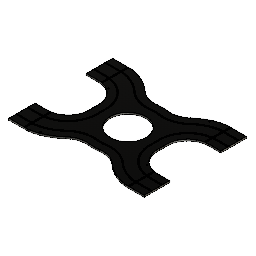
_10-16 (Round-about).bfac9250-3655-4f17-af9d-ce13ce2a29ba (Autodesk Fusion 360 design; units mm, degrees)
Autodesk Fusion 360 part; units mm, degrees
note: some values were not read from the file. Set by a fixed rule: which sketch regions a step uses.
sketch "Sketch1" plane through (0, 0, 0) normal (0, 0, 1) x (1, 0, 0)
  line L0 (0, 0) -> (609.6, 0)
  line L1 (609.6, 0) -> (609.6, -838.2)
  line L2 (609.6, -838.2) -> (0, -838.2)
  line L3 (0, -838.2) -> (0, 0)
  line L4 (0, -838.2) -> (0, -2438.4)
  line L5 (0, -2438.4) -> (609.6, -2438.4)
  line L6 (609.6, -2438.4) -> (609.6, -3276.6)
  line L7 (609.6, -3276.6) -> (0, -3276.6)
  line L8 (0, -3276.6) -> (0, -2438.4)
  line L9 (609.6, -838.2) -> (609.6, -1638.3)
  line L10 (609.6, -1638.3) -> (1036.4572, -1638.3)
  circle A0 centre (2120.9, -1638.3) radius 1084.4428
  circle A1 centre (2120.9, -1638.3) radius 558.8
  line L11 (2120.9, -1638.3) -> (3205.3428, -1638.3)
  line L12 (3205.3428, -1638.3) -> (3632.2, -1638.3)
  line L13 (2120.9, -1638.3) -> (1036.4572, -1638.3)
  line L14 (3632.2, -25.4) -> (4241.8, -25.4)
  line L15 (4241.8, -25.4) -> (4241.8, -838.2)
  line L16 (4241.8, -838.2) -> (3632.2, -838.2)
  line L17 (3632.2, -838.2) -> (3632.2, -25.4)
  line L18 (3632.2, -838.2) -> (3632.2, -2438.4)
  line L19 (3632.2, -2438.4) -> (4241.8, -2438.4)
  line L20 (4241.8, -2438.4) -> (4241.8, -3251.2)
  line L21 (4241.8, -3251.2) -> (3632.2, -3251.2)
  line L22 (3632.2, -3251.2) -> (3632.2, -2438.4)
  circle A2 centre (381.6587, -1498.6) radius 660.4
  circle A3 centre (381.6587, -1778) radius 660.4
  circle A4 centre (381.6587, -1778) radius 1515.8361
  circle A5 centre (1870.653, -3365.1042) radius 660.4
  circle A6 centre (3860.1413, -1778) radius 660.4
  circle A7 centre (3860.1413, -1498.6) radius 660.4
  circle A8 centre (3860.1413, -1778) radius 1490.7298
  circle A9 centre (2402.7721, -3360.2246) radius 660.4
  circle A10 centre (381.6587, -1498.6) radius 1515.8361
  circle A11 centre (3860.1413, -1498.6) radius 1490.7298
  circle A12 centre (1870.653, 88.5042) radius 660.4
  circle A13 centre (2402.7721, 83.6246) radius 660.4
  point P0 (3632.2, -1638.3)
  point P1 (3632.2, -1638.3)
  dimension "d1" = 609.6
  dimension "d2" = 838.2
  dimension "d3" = 1600.2
  dimension "d4" = 609.6
  dimension "d5" = 838.2
  dimension "d9" = 1117.6
  dimension "d24" = 609.6
  dimension "d36" = 1320.8
  dimension "d37" = 1320.8
  dimension "d38" = 1320.8
  dimension "d39" = 1320.8
  dimension "d40" = 1320.8
  dimension "d41" = 1320.8
  constraint horizontal L0
  constraint vertical L1
  constraint horizontal L2
  constraint vertical L3
  constraint coincident L0.start L3.end
  constraint perpendicular L2 L4
  constraint horizontal L5
  constraint vertical L6
  constraint horizontal L7
  constraint vertical L8
  constraint perpendicular L5 L9
  constraint perpendicular L9 L10
  constraint coincident L10.end A0
  constraint concentric A0 A1
  constraint coincident A0.centre A1.centre
  constraint coincident A0 L11.end
  constraint horizontal L11
  constraint parallel L11 L12
  constraint parallel L10 L13
  constraint horizontal L14
  constraint vertical L15
  constraint horizontal L16
  constraint vertical L17
  constraint perpendicular L16 L18
  constraint horizontal L19
  constraint vertical L20
  constraint horizontal L21
  constraint vertical L22
  constraint midpoint L18 P1
  constraint tangent L2 A2
  constraint tangent A0 A2
  constraint tangent A0 A3
  constraint tangent L5 A3
  constraint concentric A3 A4
  constraint coincident L6.end A4
  constraint tangent A4 A5
  constraint tangent A0 A5
  constraint tangent A0 A6
  constraint tangent L19 A6
  constraint tangent A0 A7
  constraint tangent L16 A7
  constraint concentric A6 A8
  constraint coincident L21.end A8
  constraint tangent A0 A9
  constraint tangent A8 A9
  constraint concentric A2 A10
  constraint coincident L0.end A10
  constraint concentric A7 A11
  constraint coincident L14.start A11
  constraint symmetric L11 A5 A12
  constraint symmetric L11 A9 A13
  measures "d1" distance of L0.start L0.end
  measures "d2" distance of L0.start L2.end
  measures "d3" distance of L2.end L4.end
  measures "d4" distance of L4.end L5.end
  measures "d5" distance of L4.end L7.end
  measures "d9" diameter of A1
  measures "d24" distance of L14.start L14.end
  measures "d36" diameter of A2
  measures "d37" diameter of A3
  measures "d38" diameter of A5
  measures "d39" diameter of A6
  measures "d40" diameter of A7
  measures "d41" diameter of A9
extrude "Extrude2" add sketch "Sketch1" along normal blind 50.8 contours L0 L3 A10 | L0 L1 L3 A4 A10 | L1 A0 A4 A10 | L1 L2 L3 A4 | L1 L9 A0 A2 A4 | A0 A10 A12 | L7 L8 A4 | L6 L7 L8 A4 A10 | L5 L6 L8 A10 | L2 L9 A2 | A0 A1 L13 A4 | A0 A1 A4 A10 | A0 A1 A10 A11 | L6 A0 A4 A10 | L5 L6 A0 A3 A10 | A0 A11 A13 | A0 A1 A4 A10 | A0 A1 L13 A10 | A0 A1 A8 A11 | A0 L17 A8 A11 | A0 A4 A5 | A0 A1 A4 A8 | A0 A1 L11 A8 | L14 L15 L17 A8 A11 | A0 L17 L18 A7 A8 | A0 A1 L11 A11 | A0 A1 A8 A11 | L14 L15 A11 | L15 L16 L17 A8 | A0 A8 A9 | A0 L22 A8 A11 | A0 L18 L22 A6 A11 | L16 L18 A7 | L20 L21 L22 A8 A11 | L19 L20 L22 A11 | L18 L19 A6 | L20 L21 A8
sketch "Sketch2" plane through (0, 0, 0) normal (0, 0, -1) x (1, 0, 0)
  circle A0 centre (2120.9, 1638.3) radius 558.8
  arc A1 (1418.8032, 2883.482) -> (609.6, 3276.6) centre (381.6587, 1778) ccw
  line L0 (609.6, 3276.6) -> (0, 3276.6)
  line L1 (0, 3276.6) -> (0, 2438.4)
  line L2 (0, 2438.4) -> (381.6587, 2438.4)
  arc A2 (1039.9386, 1725.1254) -> (381.6587, 2438.4) centre (381.6587, 1778) ccw
  arc A3 (1039.9386, 1725.1254) -> (1039.9386, 1551.4746) centre (2120.9, 1638.3) ccw
  arc A4 (381.6587, 838.2) -> (1039.9386, 1551.4746) centre (381.6587, 1498.6) ccw
  line L3 (381.6587, 838.2) -> (0, 838.2)
  line L4 (0, 838.2) -> (0, 0)
  line L5 (0, 0) -> (609.6, 0)
  arc A5 (609.6, 0) -> (1418.8032, 393.118) centre (381.6587, 1498.6) ccw
  arc A6 (1965.3682, 565.0685) -> (1418.8032, 393.118) centre (1870.653, -88.5042) ccw
  arc A7 (1965.3682, 565.0685) -> (2296.0872, 568.1012) centre (2120.9, 1638.3) ccw
  arc A8 (2850.1866, 402.1207) -> (2296.0872, 568.1012) centre (2402.7721, -83.6246) ccw
  arc A9 (2850.1866, 402.1207) -> (3632.2, 25.4) centre (3860.1413, 1498.6) ccw
  line L6 (3632.2, 25.4) -> (4241.8, 25.4)
  line L7 (4241.8, 25.4) -> (4241.8, 838.2)
  line L8 (4241.8, 838.2) -> (3860.1413, 838.2)
  arc A10 (3201.8614, 1551.4746) -> (3860.1413, 838.2) centre (3860.1413, 1498.6) ccw
  arc A11 (3201.8614, 1551.4746) -> (3201.8614, 1725.1254) centre (2120.9, 1638.3) ccw
  arc A12 (3860.1413, 2438.4) -> (3201.8614, 1725.1254) centre (3860.1413, 1778) ccw
  line L9 (3860.1413, 2438.4) -> (4241.8, 2438.4)
  line L10 (4241.8, 2438.4) -> (4241.8, 3251.2)
  line L11 (4241.8, 3251.2) -> (3632.2, 3251.2)
  arc A13 (3632.2, 3251.2) -> (2850.1866, 2874.4793) centre (3860.1413, 1778) ccw
  arc A14 (2296.0872, 2708.4988) -> (2850.1866, 2874.4793) centre (2402.7721, 3360.2246) ccw
  arc A15 (2296.0872, 2708.4988) -> (1965.3682, 2711.5315) centre (2120.9, 1638.3) ccw
  arc A16 (1418.8032, 2883.482) -> (1965.3682, 2711.5315) centre (1870.653, 3365.1042) ccw
  line L12 (198.4059, 2636.3069) -> (672.8085, 2636.3069) construction
  line L13 (672.8085, 2636.3069) -> (672.8085, 3106.5481) construction
  line L14 (672.8085, 3106.5481) -> (198.4059, 3106.5481) construction
  line L15 (198.4059, 3106.5481) -> (198.4059, 2636.3069) construction
  line L16 (0, 508) -> (482.6, 508)
  line L17 (0, 2794) -> (482.6, 2794)
  line L18 (4241.8, 272.4179) -> (3759.2, 272.4179)
  line L19 (4241.8, 2844.8) -> (3759.2, 2844.8)
  line L20 (482.6, 508) -> (482.6, 0)
  line L21 (3759.2, 272.4179) -> (3759.2, 845.96)
  line L22 (3759.2, 2844.8) -> (3759.2, 2430.64)
  line L23 (482.6, 2794) -> (482.6, 2430.64)
  line L24 (482.6, 2430.64) -> (511.175, 2430.64)
  line L25 (511.175, 2430.64) -> (511.175, 3276.6)
  line L26 (511.175, 3276.6) -> (482.6, 3276.6)
  line L27 (482.6, 3276.6) -> (482.6, 2430.64)
  line L28 (482.6, 0) -> (511.175, 0)
  line L29 (511.175, 0) -> (511.175, 851.0248)
  line L30 (511.175, 851.0248) -> (482.6, 851.0248)
  line L31 (482.6, 851.0248) -> (482.6, 0)
  line L32 (3759.2, 845.96) -> (3730.625, 845.96)
  line L33 (3730.625, 845.96) -> (3730.625, 25.4)
  line L34 (3730.625, 25.4) -> (3759.2, 25.4)
  line L35 (3759.2, 25.4) -> (3759.2, 845.96)
  line L36 (3759.2, 2430.64) -> (3730.625, 2430.64)
  line L37 (3730.625, 2430.64) -> (3730.625, 3251.2)
  line L38 (3730.625, 3251.2) -> (3759.2, 3251.2)
  line L39 (3759.2, 3251.2) -> (3759.2, 2430.64)
  dimension "d44" = 254
  dimension "d45" = 482.6
  dimension "d46" = 482.6
  dimension "d47" = 482.6
  dimension "d48" = 482.6
  dimension "d49" = 28.575
  dimension "d50" = 28.575
  dimension "d51" = 28.575
  constraint coincident L4 L16.start
  constraint perpendicular L4 L16
  constraint coincident L1 L17.start
  constraint perpendicular L15 L17
  constraint coincident L7 L18.start
  constraint perpendicular L7 L18
  constraint midpoint L10 L19.start
  constraint perpendicular L10 L19
  constraint coincident L5 L20.end
  constraint perpendicular L5 L20
  constraint coincident A10 L21.end
  constraint perpendicular L18 L21
  constraint coincident A12 L22.end
  constraint perpendicular L19 L22
  constraint coincident A2 L23.end
  constraint perpendicular L2 L23
  constraint horizontal L24
  constraint vertical L25
  constraint horizontal L26
  constraint vertical L27
  constraint coincident L0 L25.end
  constraint horizontal L28
  constraint vertical L29
  constraint horizontal L30
  constraint vertical L31
  constraint coincident A4 L29.end
  constraint horizontal L32
  constraint vertical L33
  constraint horizontal L34
  constraint vertical L35
  constraint coincident L6 L33.end
  constraint horizontal L36
  constraint vertical L37
  constraint horizontal L38
  constraint vertical L39
  constraint coincident L11 L37.end
  measures "d45" distance of L16.start L16.end
  measures "d46" distance of L17.start L17.end
  measures "d47" distance of L18.start L18.end
  measures "d48" distance of L19.start L19.end
  measures "d49" distance of L23.end L24.end
  measures "d50" distance of L21.end L32.end
  measures "d51" distance of L22.end L36.end
extrude "Extrude3" add sketch "Sketch2" against normal blind 50.8254 contours L0 L23 L24 L25 L26 L27 | L11 L22 L36 L37 L38 L39 | A4 L5 L20 L28 L29 L31 | L6 L21 L32 L33 L34 L35
sketch "Sketch3" plane through (0, 0, 50.8) normal (0, 0, 1) x (-1, 0, 0)
  line L0 (-511.175, 2430.64) -> (-511.175, 3276.6)
  line L1 (-511.175, 3276.6) -> (-609.6, 3276.6)
  arc A0 (-609.6, 3276.6) -> (-1418.8032, 2883.482) centre (-381.6587, 1778) ccw
  arc A1 (-1965.3682, 2711.5315) -> (-1418.8032, 2883.482) centre (-1870.653, 3365.1042) ccw
  arc A2 (-1965.3682, 2711.5315) -> (-2296.0872, 2708.4988) centre (-2120.9, 1638.3) ccw
  arc A3 (-2850.1866, 2874.4793) -> (-2296.0872, 2708.4988) centre (-2402.7721, 3360.2246) ccw
  arc A4 (-2850.1866, 2874.4793) -> (-3632.2, 3251.2) centre (-3860.1413, 1778) ccw
  line L2 (-3632.2, 3251.2) -> (-3730.625, 3251.2)
  line L3 (-3730.625, 3251.2) -> (-3730.625, 2430.64)
  line L4 (-3730.625, 2430.64) -> (-3759.2, 2430.64)
  arc A5 (-3201.8614, 1725.1254) -> (-3759.2, 2430.64) centre (-3860.1413, 1778) ccw
  arc A6 (-3201.8614, 1725.1254) -> (-3201.8614, 1551.4746) centre (-2120.9, 1638.3) ccw
  arc A7 (-3759.2, 845.96) -> (-3201.8614, 1551.4746) centre (-3860.1413, 1498.6) ccw
  line L5 (-3759.2, 845.96) -> (-3730.625, 845.96)
  line L6 (-3730.625, 845.96) -> (-3730.625, 25.4)
  line L7 (-3730.625, 25.4) -> (-3632.2, 25.4)
  arc A8 (-3632.2, 25.4) -> (-2850.1866, 402.1207) centre (-3860.1413, 1498.6) ccw
  arc A9 (-2296.0872, 568.1012) -> (-2850.1866, 402.1207) centre (-2402.7721, -83.6246) ccw
  arc A10 (-2296.0872, 568.1012) -> (-1965.3682, 565.0685) centre (-2120.9, 1638.3) ccw
  arc A11 (-1418.8032, 393.118) -> (-1965.3682, 565.0685) centre (-1870.653, -88.5042) ccw
  arc A12 (-1418.8032, 393.118) -> (-609.6, 0) centre (-381.6587, 1498.6) ccw
  line L8 (-609.6, 0) -> (-511.175, 0)
  line L9 (-511.175, 0) -> (-511.175, 851.0248)
  arc A13 (-1039.9386, 1551.4746) -> (-511.175, 851.0248) centre (-381.6587, 1498.6) ccw
  arc A14 (-1039.9386, 1551.4746) -> (-1039.9386, 1725.1254) centre (-2120.9, 1638.3) ccw
  arc A15 (-482.6, 2430.64) -> (-1039.9386, 1725.1254) centre (-381.6587, 1778) ccw
  line L10 (-482.6, 2430.64) -> (-511.175, 2430.64)
  circle A16 centre (-2120.9, 1638.3) radius 558.8
  line L11 (-568.325, 57.15) -> (-568.325, 805.7553)
  arc A17 (-1096.9052, 1556.0503) -> (-568.325, 805.7553) centre (-381.6587, 1498.6) ccw
  arc A18 (-1096.9052, 1556.0503) -> (-1096.9052, 1720.5497) centre (-2120.9, 1638.3) ccw
  arc A19 (-568.325, 2470.8447) -> (-1096.9052, 1720.5497) centre (-381.6587, 1778) ccw
  line L12 (-568.325, 2470.8447) -> (-568.325, 3219.45)
  line L13 (-568.325, 3219.45) -> (-605.2368, 3219.45)
  arc A20 (-605.2368, 3219.45) -> (-1379.7009, 2841.8032) centre (-381.6587, 1778) ccw
  arc A21 (-1973.5647, 2654.9724) -> (-1379.7009, 2841.8032) centre (-1870.653, 3365.1042) ccw
  arc A22 (-1973.5647, 2654.9724) -> (-2286.8549, 2652.0995) centre (-2120.9, 1638.3) ccw
  arc A23 (-2888.9051, 2832.4437) -> (-2286.8549, 2652.0995) centre (-2402.7721, 3360.2246) ccw
  arc A24 (-2888.9051, 2832.4437) -> (-3636.6383, 3194.05) centre (-3860.1413, 1778) ccw
  line L14 (-3636.6383, 3194.05) -> (-3673.475, 3194.05)
  line L15 (-3673.475, 3194.05) -> (-3673.475, 2470.8447)
  arc A25 (-3144.8948, 1720.5497) -> (-3673.475, 2470.8447) centre (-3860.1413, 1778) ccw
  arc A26 (-3144.8948, 1720.5497) -> (-3144.8948, 1556.0503) centre (-2120.9, 1638.3) ccw
  arc A27 (-3673.475, 805.7553) -> (-3144.8948, 1556.0503) centre (-3860.1413, 1498.6) ccw
  line L16 (-3673.475, 805.7553) -> (-3673.475, 82.55)
  line L17 (-3673.475, 82.55) -> (-3636.6383, 82.55)
  arc A28 (-3636.6383, 82.55) -> (-2888.9051, 444.1563) centre (-3860.1413, 1498.6) ccw
  arc A29 (-2286.8549, 624.5005) -> (-2888.9051, 444.1563) centre (-2402.7721, -83.6246) ccw
  arc A30 (-2286.8549, 624.5005) -> (-1973.5647, 621.6276) centre (-2120.9, 1638.3) ccw
  arc A31 (-1379.7009, 434.7968) -> (-1973.5647, 621.6276) centre (-1870.653, -88.5042) ccw
  arc A32 (-1379.7009, 434.7968) -> (-605.2368, 57.15) centre (-381.6587, 1498.6) ccw
  line L18 (-605.2368, 57.15) -> (-568.325, 57.15)
  circle A33 centre (-762, 890.1441) radius 16
  line L19 (-4241.8, 838.2) -> (-4241.8, 25.4)
  circle A34 centre (-3251.2, 200.7781) radius 16
  line L20 (-4241.8, 3251.2) -> (-4241.8, 2438.4)
  line L21 (0, 2438.4) -> (0, 3276.6)
  circle A35 centre (-3454.4, 2369.8209) radius 16
  line L22 (0, 2857.5) -> (-876.3, 2857.5)
  line L23 (-876.3, 2857.5) -> (-876.3, 3150.2592)
  circle A36 centre (-876.3, 3150.2592) radius 16
  circle A37 centre (-2120.9, 1638.3) radius 559.8
  dimension "d54" = -57.15
  dimension "d56" = 32
  dimension "d58" = 32
  dimension "d60" = 32
  dimension "d61" = 876.3
  dimension "d62" = 32
  dimension "d63" = 1
  constraint midpoint L21 L22.start
  constraint perpendicular L12 L22
  constraint coincident A20 L23.end
  constraint perpendicular L22 L23
  constraint coincident L23.end A36.centre
  measures "d56" diameter of A33
  measures "d58" diameter of A34
  measures "d60" diameter of A35
  measures "d61" distance of L22.start L22.end
  measures "d62" diameter of A36
extrude "Extrude4" add sketch "Sketch3" along normal blind 0.0254 contours A17 A33 | A17 A33 | A28 A34 | A28 A34 | A20 L23 A36 | A20 L23 A36 | A20 A36 | A25 A35 | A25 A35
sketch "Sketch4" plane through (0, 0, 50.8) normal (0, 0, 1) x (-1, 0, 0)
  line L0 (-482.6, 845.96) -> (-482.6, 0)
  line L1 (-482.6, 0) -> (0, 0)
  line L2 (0, 0) -> (0, 838.2)
  line L3 (0, 838.2) -> (-381.6587, 838.2)
  arc A0 (-482.6, 845.96) -> (-381.6587, 838.2) centre (-381.6587, 1498.6) ccw
  line L4 (0, 587.375) -> (-381.6587, 587.375)
  arc A1 (-520.9383, 598.0823) -> (-381.6587, 587.375) centre (-381.6587, 1498.6) ccw
  line L5 (0, 606.425) -> (-381.6587, 606.425)
  arc A2 (-518.0265, 616.9084) -> (-381.6587, 606.425) centre (-381.6587, 1498.6) ccw
  dimension "d66" = 250.825
  dimension "d67" = 231.775
extrude "Extrude5" add sketch "Sketch4" along normal blind 0.0279 contours L0 L2 L4 A1 L5 A2
sketch "Sketch5" plane through (0, 0, 50.8) normal (0, 0, 1) x (-1, 0, 0)
  line L0 (0, 587.375) -> (-381.6587, 587.375)
  arc A0 (-482.6, 592.9832) -> (-381.6587, 587.375) centre (-381.6587, 1498.6) ccw
  line L1 (-482.6, 592.9832) -> (-482.6, 0)
  line L2 (-482.6, 0) -> (0, 0)
  line L3 (0, 0) -> (0, 587.375)
  line L4 (-482.6, 250.825) -> (0, 250.825)
  line L5 (-482.6, 231.775) -> (0, 231.775)
  dimension "d70" = -250.825
  dimension "d71" = -231.775
extrude "Extrude6" add sketch "Sketch5" along normal blind 0.0279 contours L1 L3 L4 L5
sketch "Sketch6" plane through (0, 0, 50.8) normal (0, 0, 1) x (-1, 0, 0)
  circle A0 centre (-762, 890.1441) radius 16
  circle A1 centre (-876.3, 3150.2592) radius 16
  circle A2 centre (-3251.2, 200.7781) radius 16
  circle A3 centre (-3454.4, 2369.8209) radius 16
  line L0 (-511.175, 2430.64) -> (-511.175, 3276.6)
  line L1 (-511.175, 3276.6) -> (-609.6, 3276.6)
  arc A4 (-609.6, 3276.6) -> (-1418.8032, 2883.482) centre (-381.6587, 1778) ccw
  arc A5 (-1965.3682, 2711.5315) -> (-1418.8032, 2883.482) centre (-1870.653, 3365.1042) ccw
  arc A6 (-1965.3682, 2711.5315) -> (-2296.0872, 2708.4988) centre (-2120.9, 1638.3) ccw
  arc A7 (-2850.1866, 2874.4793) -> (-2296.0872, 2708.4988) centre (-2402.7721, 3360.2246) ccw
  arc A8 (-2850.1866, 2874.4793) -> (-3632.2, 3251.2) centre (-3860.1413, 1778) ccw
  line L2 (-3632.2, 3251.2) -> (-3730.625, 3251.2)
  line L3 (-3730.625, 3251.2) -> (-3730.625, 2430.64)
  line L4 (-3730.625, 2430.64) -> (-3759.2, 2430.64)
  arc A9 (-3201.8614, 1725.1254) -> (-3759.2, 2430.64) centre (-3860.1413, 1778) ccw
  arc A10 (-3201.8614, 1725.1254) -> (-3201.8614, 1551.4746) centre (-2120.9, 1638.3) ccw
  arc A11 (-3759.2, 845.96) -> (-3201.8614, 1551.4746) centre (-3860.1413, 1498.6) ccw
  line L5 (-3759.2, 845.96) -> (-3730.625, 845.96)
  line L6 (-3730.625, 845.96) -> (-3730.625, 25.4)
  line L7 (-3730.625, 25.4) -> (-3632.2, 25.4)
  arc A12 (-3632.2, 25.4) -> (-2850.1866, 402.1207) centre (-3860.1413, 1498.6) ccw
  arc A13 (-2296.0872, 568.1012) -> (-2850.1866, 402.1207) centre (-2402.7721, -83.6246) ccw
  arc A14 (-2296.0872, 568.1012) -> (-1965.3682, 565.0685) centre (-2120.9, 1638.3) ccw
  arc A15 (-1418.8032, 393.118) -> (-1965.3682, 565.0685) centre (-1870.653, -88.5042) ccw
  arc A16 (-1418.8032, 393.118) -> (-609.6, 0) centre (-381.6587, 1498.6) ccw
  line L8 (-609.6, 0) -> (-511.175, 0)
  line L9 (-511.175, 0) -> (-511.175, 851.0248)
  arc A17 (-1039.9386, 1551.4746) -> (-511.175, 851.0248) centre (-381.6587, 1498.6) ccw
  arc A18 (-1039.9386, 1551.4746) -> (-1039.9386, 1725.1254) centre (-2120.9, 1638.3) ccw
  arc A19 (-482.6, 2430.64) -> (-1039.9386, 1725.1254) centre (-381.6587, 1778) ccw
  line L10 (-482.6, 2430.64) -> (-511.175, 2430.64)
  circle A20 centre (-2120.9, 1638.3) radius 558.8
  line L11 (-3730.625, 276.225) -> (-3652.3833, 276.225)
  arc A21 (-3652.3833, 276.225) -> (-3020.118, 586.6104) centre (-3860.1413, 1498.6) ccw
  arc A22 (-2255.5675, 815.6316) -> (-3020.118, 586.6104) centre (-2402.7721, -83.6246) ccw
  arc A23 (-2255.5675, 815.6316) -> (-2001.3418, 813.3004) centre (-2120.9, 1638.3) ccw
  arc A24 (-1247.1872, 576.0418) -> (-2001.3418, 813.3004) centre (-1870.653, -88.5042) ccw
  arc A25 (-1247.1872, 576.0418) -> (-589.771, 250.825) centre (-381.6587, 1498.6) ccw
  line L12 (-589.771, 250.825) -> (-511.175, 250.825)
  line L13 (-3730.625, 257.175) -> (-3650.7821, 257.175)
  arc A26 (-3650.7821, 257.175) -> (-3007.2118, 572.5986) centre (-3860.1413, 1498.6) ccw
  arc A27 (-2258.6449, 796.8319) -> (-3007.2118, 572.5986) centre (-2402.7721, -83.6246) ccw
  arc A28 (-2258.6449, 796.8319) -> (-1998.6096, 794.4473) centre (-2120.9, 1638.3) ccw
  arc A29 (-1260.2214, 562.1489) -> (-1998.6096, 794.4473) centre (-1870.653, -88.5042) ccw
  arc A30 (-1260.2214, 562.1489) -> (-591.3428, 231.775) centre (-381.6587, 1498.6) ccw
  line L14 (-591.3428, 231.775) -> (-511.175, 231.775)
  dimension "d74" = -250.825
  dimension "d75" = -231.775
extrude "Extrude7" add sketch "Sketch6" along normal blind 0.0279 contours L6 L9 L11 A21 A22 A23 A24 A25 L12 L13 A26 A27 A28 A29 A30 L14
sketch "Sketch7" plane through (0, 0, 50.8) normal (0, 0, 1) x (-1, 0, 0)
  circle A0 centre (-2120.9, 1638.3) radius 558.8
  line L0 (-3730.625, 276.225) -> (-3652.3833, 276.225)
  arc A1 (-3652.3833, 276.225) -> (-3020.118, 586.6104) centre (-3860.1413, 1498.6) ccw
  arc A2 (-2255.5675, 815.6316) -> (-3020.118, 586.6104) centre (-2402.7721, -83.6246) ccw
  arc A3 (-2255.5675, 815.6316) -> (-2001.3418, 813.3004) centre (-2120.9, 1638.3) ccw
  arc A4 (-1247.1872, 576.0418) -> (-2001.3418, 813.3004) centre (-1870.653, -88.5042) ccw
  arc A5 (-1247.1872, 576.0418) -> (-589.771, 250.825) centre (-381.6587, 1498.6) ccw
  line L1 (-589.771, 250.825) -> (-511.175, 250.825)
  line L2 (-511.175, 250.825) -> (-511.175, 851.0248)
  arc A6 (-1039.9386, 1551.4746) -> (-511.175, 851.0248) centre (-381.6587, 1498.6) ccw
  arc A7 (-1039.9386, 1551.4746) -> (-1039.9386, 1725.1254) centre (-2120.9, 1638.3) ccw
  arc A8 (-482.6, 2430.64) -> (-1039.9386, 1725.1254) centre (-381.6587, 1778) ccw
  line L3 (-482.6, 2430.64) -> (-511.175, 2430.64)
  line L4 (-511.175, 2430.64) -> (-511.175, 3276.6)
  line L5 (-511.175, 3276.6) -> (-609.6, 3276.6)
  arc A9 (-609.6, 3276.6) -> (-1418.8032, 2883.482) centre (-381.6587, 1778) ccw
  arc A10 (-1965.3682, 2711.5315) -> (-1418.8032, 2883.482) centre (-1870.653, 3365.1042) ccw
  arc A11 (-1965.3682, 2711.5315) -> (-2296.0872, 2708.4988) centre (-2120.9, 1638.3) ccw
  arc A12 (-2850.1866, 2874.4793) -> (-2296.0872, 2708.4988) centre (-2402.7721, 3360.2246) ccw
  arc A13 (-2850.1866, 2874.4793) -> (-3632.2, 3251.2) centre (-3860.1413, 1778) ccw
  line L6 (-3632.2, 3251.2) -> (-3730.625, 3251.2)
  line L7 (-3730.625, 3251.2) -> (-3730.625, 2430.64)
  line L8 (-3730.625, 2430.64) -> (-3759.2, 2430.64)
  arc A14 (-3201.8614, 1725.1254) -> (-3759.2, 2430.64) centre (-3860.1413, 1778) ccw
  arc A15 (-3201.8614, 1725.1254) -> (-3201.8614, 1551.4746) centre (-2120.9, 1638.3) ccw
  arc A16 (-3759.2, 845.96) -> (-3201.8614, 1551.4746) centre (-3860.1413, 1498.6) ccw
  line L9 (-3759.2, 845.96) -> (-3730.625, 845.96)
  line L10 (-3730.625, 845.96) -> (-3730.625, 276.225)
  circle A17 centre (-3454.4, 2369.8209) radius 16
  circle A18 centre (-876.3, 3150.2592) radius 16
  circle A19 centre (-762, 890.1441) radius 16
  arc A20 (-1289.9584, 1571.5568) -> (-560.3663, 605.0707) centre (-381.6587, 1498.6) ccw
  arc A21 (-1270.9696, 1570.0316) -> (-556.6302, 623.7507) centre (-381.6587, 1498.6) ccw
  line L11 (-556.6302, 623.7507) -> (-511.175, 614.6596)
  line L12 (-560.3663, 605.0707) -> (-511.175, 595.2323)
  arc A22 (-1289.9584, 1571.5568) -> (-1289.9584, 1705.0432) centre (-2120.9, 1638.3) ccw
  arc A23 (-1270.9696, 1570.0316) -> (-1270.9696, 1706.5684) centre (-2120.9, 1638.3) ccw
  arc A24 (-520.9383, 2678.5177) -> (-1289.9584, 1705.0432) centre (-381.6587, 1778) ccw
  arc A25 (-518.0265, 2659.6916) -> (-1270.9696, 1706.5684) centre (-381.6587, 1778) ccw
  line L13 (-518.0265, 2659.6916) -> (-511.175, 2660.7513)
  line L14 (-520.9383, 2678.5177) -> (-511.175, 2680.0278)
  dimension "d78" = 250.825
  dimension "d79" = 231.775
  dimension "d80" = -250.825
  dimension "d81" = -231.775
  dimension "d82" = 250.825
  dimension "d83" = 231.775
  constraint coincident L2 L11.end
  constraint tangent A21 L11
  constraint coincident L2 L12.end
  constraint tangent A20 L12
  constraint coincident L4 L13.end
  constraint tangent A25 L13
  constraint coincident L4 L14.end
  constraint tangent A24 L14
extrude "Extrude8" add sketch "Sketch7" along normal blind 0.0279 contours L2 L4 A20 A21 L11 L12 A22 A23 A24 A25 L13 L14
sketch "Sketch8" plane through (0, 0, 50.8) normal (0, 0, 1) x (-1, 0, 0)
  line L0 (-482.6, 3276.6) -> (-482.6, 2430.64)
  arc A0 (-381.6587, 2438.4) -> (-482.6, 2430.64) centre (-381.6587, 1778) ccw
  line L1 (-381.6587, 2438.4) -> (0, 2438.4)
  line L2 (0, 2438.4) -> (0, 3276.6)
  line L3 (0, 3276.6) -> (-482.6, 3276.6)
  line L4 (-381.6587, 2689.225) -> (0, 2689.225)
  arc A1 (-381.6587, 2689.225) -> (-520.9383, 2678.5177) centre (-381.6587, 1778) ccw
  line L5 (-381.6587, 2670.175) -> (0, 2670.175)
  arc A2 (-381.6587, 2670.175) -> (-518.0265, 2659.6916) centre (-381.6587, 1778) ccw
  line L6 (0, 3025.775) -> (-482.6, 3025.775)
  line L7 (0, 3044.825) -> (-482.6, 3044.825)
  dimension "d86" = 250.825
  dimension "d87" = 231.775
  dimension "d88" = -250.825
  dimension "d89" = -231.775
extrude "Extrude9" add sketch "Sketch8" along normal blind 0.0279 contours L0 L2 L4 A1 L5 A2
extrude "Extrude10" add sketch "Sketch8" along normal blind 0.0279 contours L0 L2 L6 L7
sketch "Sketch9" plane through (0, 0, 50.8) normal (0, 0, 1) x (-1, 0, 0)
  line L0 (-520.9383, 2678.5177) -> (-511.175, 2680.0278)
  line L1 (-511.175, 2680.0278) -> (-511.175, 3276.6)
  line L2 (-511.175, 3276.6) -> (-609.6, 3276.6)
  arc A0 (-609.6, 3276.6) -> (-1418.8032, 2883.482) centre (-381.6587, 1778) ccw
  arc A1 (-1965.3682, 2711.5315) -> (-1418.8032, 2883.482) centre (-1870.653, 3365.1042) ccw
  arc A2 (-1965.3682, 2711.5315) -> (-2296.0872, 2708.4988) centre (-2120.9, 1638.3) ccw
  arc A3 (-2850.1866, 2874.4793) -> (-2296.0872, 2708.4988) centre (-2402.7721, 3360.2246) ccw
  arc A4 (-2850.1866, 2874.4793) -> (-3632.2, 3251.2) centre (-3860.1413, 1778) ccw
  line L3 (-3632.2, 3251.2) -> (-3730.625, 3251.2)
  line L4 (-3730.625, 3251.2) -> (-3730.625, 2430.64)
  line L5 (-3730.625, 2430.64) -> (-3759.2, 2430.64)
  arc A5 (-3201.8614, 1725.1254) -> (-3759.2, 2430.64) centre (-3860.1413, 1778) ccw
  arc A6 (-3201.8614, 1725.1254) -> (-3201.8614, 1551.4746) centre (-2120.9, 1638.3) ccw
  arc A7 (-3759.2, 845.96) -> (-3201.8614, 1551.4746) centre (-3860.1413, 1498.6) ccw
  line L6 (-3759.2, 845.96) -> (-3730.625, 845.96)
  line L7 (-3730.625, 845.96) -> (-3730.625, 276.225)
  line L8 (-3730.625, 276.225) -> (-3652.3833, 276.225)
  arc A8 (-3652.3833, 276.225) -> (-3020.118, 586.6104) centre (-3860.1413, 1498.6) ccw
  arc A9 (-2255.5675, 815.6316) -> (-3020.118, 586.6104) centre (-2402.7721, -83.6246) ccw
  arc A10 (-2255.5675, 815.6316) -> (-2001.3418, 813.3004) centre (-2120.9, 1638.3) ccw
  arc A11 (-1247.1872, 576.0418) -> (-2001.3418, 813.3004) centre (-1870.653, -88.5042) ccw
  arc A12 (-1247.1872, 576.0418) -> (-589.771, 250.825) centre (-381.6587, 1498.6) ccw
  line L9 (-589.771, 250.825) -> (-511.175, 250.825)
  line L10 (-511.175, 250.825) -> (-511.175, 595.2323)
  line L11 (-511.175, 595.2323) -> (-560.3663, 605.0707)
  arc A13 (-1289.9584, 1571.5568) -> (-560.3663, 605.0707) centre (-381.6587, 1498.6) ccw
  arc A14 (-1289.9584, 1571.5568) -> (-1289.9584, 1705.0432) centre (-2120.9, 1638.3) ccw
  arc A15 (-520.9383, 2678.5177) -> (-1289.9584, 1705.0432) centre (-381.6587, 1778) ccw
  circle A16 centre (-2120.9, 1638.3) radius 558.8
  circle A17 centre (-3454.4, 2369.8209) radius 16
  circle A18 centre (-876.3, 3150.2592) radius 16
  line L12 (-511.175, 3025.775) -> (-589.771, 3025.775)
  arc A19 (-589.771, 3025.775) -> (-1247.1872, 2700.5582) centre (-381.6587, 1778) ccw
  arc A20 (-2001.3418, 2463.2996) -> (-1247.1872, 2700.5582) centre (-1870.653, 3365.1042) ccw
  arc A21 (-2001.3418, 2463.2996) -> (-2255.5675, 2460.9684) centre (-2120.9, 1638.3) ccw
  arc A22 (-3020.118, 2689.9896) -> (-2255.5675, 2460.9684) centre (-2402.7721, 3360.2246) ccw
  arc A23 (-3020.118, 2689.9896) -> (-3652.3833, 3000.375) centre (-3860.1413, 1778) ccw
  line L13 (-3652.3833, 3000.375) -> (-3730.625, 3000.375)
  line L14 (-511.175, 3044.825) -> (-591.3428, 3044.825)
  arc A24 (-591.3428, 3044.825) -> (-1260.2214, 2714.4511) centre (-381.6587, 1778) ccw
  arc A25 (-1998.6096, 2482.1527) -> (-1260.2214, 2714.4511) centre (-1870.653, 3365.1042) ccw
  arc A26 (-1998.6096, 2482.1527) -> (-2258.6449, 2479.7681) centre (-2120.9, 1638.3) ccw
  arc A27 (-3007.2118, 2704.0014) -> (-2258.6449, 2479.7681) centre (-2402.7721, 3360.2246) ccw
  arc A28 (-3007.2118, 2704.0014) -> (-3650.7821, 3019.425) centre (-3860.1413, 1778) ccw
  line L15 (-3650.7821, 3019.425) -> (-3730.625, 3019.425)
  dimension "d94" = -250.825
  dimension "d95" = -231.775
extrude "Extrude11" add sketch "Sketch9" along normal blind 0.0279 contours L1 L4 L12 A19 A20 A21 A22 A23 L13 L14 A24 A25 A26 A27 A28 L15
sketch "Sketch10" plane through (0, 0, 50.8) normal (0, 0, 1) x (-1, 0, 0)
  line L0 (-3652.3833, 3000.375) -> (-3730.625, 3000.375)
  line L1 (-3730.625, 3000.375) -> (-3730.625, 2430.64)
  line L2 (-3730.625, 2430.64) -> (-3759.2, 2430.64)
  arc A0 (-3201.8614, 1725.1254) -> (-3759.2, 2430.64) centre (-3860.1413, 1778) ccw
  arc A1 (-3201.8614, 1725.1254) -> (-3201.8614, 1551.4746) centre (-2120.9, 1638.3) ccw
  arc A2 (-3759.2, 845.96) -> (-3201.8614, 1551.4746) centre (-3860.1413, 1498.6) ccw
  line L3 (-3759.2, 845.96) -> (-3730.625, 845.96)
  line L4 (-3730.625, 845.96) -> (-3730.625, 276.225)
  line L5 (-3730.625, 276.225) -> (-3652.3833, 276.225)
  arc A3 (-3652.3833, 276.225) -> (-3020.118, 586.6104) centre (-3860.1413, 1498.6) ccw
  arc A4 (-2255.5675, 815.6316) -> (-3020.118, 586.6104) centre (-2402.7721, -83.6246) ccw
  arc A5 (-2255.5675, 815.6316) -> (-2001.3418, 813.3004) centre (-2120.9, 1638.3) ccw
  arc A6 (-1247.1872, 576.0418) -> (-2001.3418, 813.3004) centre (-1870.653, -88.5042) ccw
  arc A7 (-1247.1872, 576.0418) -> (-589.771, 250.825) centre (-381.6587, 1498.6) ccw
  line L6 (-589.771, 250.825) -> (-511.175, 250.825)
  line L7 (-511.175, 250.825) -> (-511.175, 595.2323)
  line L8 (-511.175, 595.2323) -> (-560.3663, 605.0707)
  arc A8 (-1289.9584, 1571.5568) -> (-560.3663, 605.0707) centre (-381.6587, 1498.6) ccw
  arc A9 (-1289.9584, 1571.5568) -> (-1289.9584, 1705.0432) centre (-2120.9, 1638.3) ccw
  arc A10 (-520.9383, 2678.5177) -> (-1289.9584, 1705.0432) centre (-381.6587, 1778) ccw
  line L9 (-520.9383, 2678.5177) -> (-511.175, 2680.0278)
  line L10 (-511.175, 2680.0278) -> (-511.175, 3025.775)
  line L11 (-511.175, 3025.775) -> (-589.771, 3025.775)
  arc A11 (-589.771, 3025.775) -> (-1247.1872, 2700.5582) centre (-381.6587, 1778) ccw
  arc A12 (-2001.3418, 2463.2996) -> (-1247.1872, 2700.5582) centre (-1870.653, 3365.1042) ccw
  arc A13 (-2001.3418, 2463.2996) -> (-2255.5675, 2460.9684) centre (-2120.9, 1638.3) ccw
  arc A14 (-3020.118, 2689.9896) -> (-2255.5675, 2460.9684) centre (-2402.7721, 3360.2246) ccw
  arc A15 (-3020.118, 2689.9896) -> (-3652.3833, 3000.375) centre (-3860.1413, 1778) ccw
  circle A16 centre (-2120.9, 1638.3) radius 558.8
  circle A17 centre (-3454.4, 2369.8209) radius 16
  arc A18 (-3720.8617, 598.0823) -> (-2951.8416, 1571.5568) centre (-3860.1413, 1498.6) ccw
  arc A19 (-2951.8416, 1705.0432) -> (-2951.8416, 1571.5568) centre (-2120.9, 1638.3) ccw
  arc A20 (-2951.8416, 1705.0432) -> (-3720.8617, 2678.5177) centre (-3860.1413, 1778) ccw
  arc A21 (-3723.7735, 616.9084) -> (-2970.8304, 1570.0316) centre (-3860.1413, 1498.6) ccw
  arc A22 (-2970.8304, 1706.5684) -> (-2970.8304, 1570.0316) centre (-2120.9, 1638.3) ccw
  arc A23 (-2970.8304, 1706.5684) -> (-3723.7735, 2659.6916) centre (-3860.1413, 1778) ccw
  line L12 (-3720.8617, 598.0823) -> (-3730.625, 596.5722)
  line L13 (-3723.7735, 616.9084) -> (-3730.625, 615.8487)
  line L14 (-3723.7735, 2659.6916) -> (-3730.625, 2660.7513)
  line L15 (-3720.8617, 2678.5177) -> (-3730.625, 2680.0278)
  dimension "d98" = 250.825
  dimension "d99" = 231.775
  constraint coincident L4 L12.end
  constraint tangent A18 L12
  constraint coincident L4 L13.end
  constraint tangent A21 L13
  constraint coincident L1 L14.end
  constraint tangent A23 L14
  constraint coincident L1 L15.end
  constraint tangent A20 L15
extrude "Extrude12" add sketch "Sketch10" along normal blind 0.0279 contours L1 L4 A18 A19 A20 A21 A22 A23 L12 L13 L14 L15
sketch "Sketch11" plane through (0, 0, 50.8) normal (0, 0, 1) x (-1, 0, 0)
  line L0 (-3759.2, 2430.64) -> (-3759.2, 3251.2)
  line L1 (-3759.2, 3251.2) -> (-4241.8, 3251.2)
  line L2 (-4241.8, 3251.2) -> (-4241.8, 2438.4)
  line L3 (-4241.8, 2438.4) -> (-3860.1413, 2438.4)
  arc A0 (-3759.2, 2430.64) -> (-3860.1413, 2438.4) centre (-3860.1413, 1778) ccw
  line L4 (-4241.8, 2689.225) -> (-3860.1413, 2689.225)
  arc A1 (-3720.8617, 2678.5177) -> (-3860.1413, 2689.225) centre (-3860.1413, 1778) ccw
  arc A2 (-3723.7735, 2659.6916) -> (-3860.1413, 2670.175) centre (-3860.1413, 1778) ccw
  line L5 (-4241.8, 2670.175) -> (-3860.1413, 2670.175)
  dimension "d103" = -231.775
extrude "Extrude13" add sketch "Sketch11" along normal blind 0.0279 contours L0 L2 L4 A1 A2 L5
sketch "Sketch12" plane through (0, 0, 50.8) normal (0, 0, 1) x (-1, 0, 0)
  line L0 (-4241.8, 2689.225) -> (-3860.1413, 2689.225)
  arc A0 (-3759.2, 2683.6168) -> (-3860.1413, 2689.225) centre (-3860.1413, 1778) ccw
  line L1 (-3759.2, 2683.6168) -> (-3759.2, 3251.2)
  line L2 (-3759.2, 3251.2) -> (-4241.8, 3251.2)
  line L3 (-4241.8, 3251.2) -> (-4241.8, 2689.225)
  line L4 (-3759.2, 3000.375) -> (-4241.8, 3000.375)
  line L5 (-3759.2, 3019.425) -> (-4241.8, 3019.425)
  dimension "d106" = -250.825
  dimension "d107" = -231.775
extrude "Extrude14" add sketch "Sketch12" along normal blind 0.0279 contours L1 L3 L4 L5
sketch "Sketch13" plane through (0, 0, 50.8) normal (0, 0, 1) x (-1, 0, 0)
  line L0 (-3759.2, 25.4) -> (-3759.2, 845.96)
  arc A0 (-3860.1413, 838.2) -> (-3759.2, 845.96) centre (-3860.1413, 1498.6) ccw
  line L1 (-3860.1413, 838.2) -> (-4241.8, 838.2)
  line L2 (-4241.8, 838.2) -> (-4241.8, 25.4)
  line L3 (-4241.8, 25.4) -> (-3759.2, 25.4)
  line L4 (-4241.8, 276.225) -> (-3759.2, 276.225)
  line L5 (-4241.8, 257.175) -> (-3759.2, 257.175)
  line L6 (-3860.1413, 587.375) -> (-4241.8, 587.375)
  arc A1 (-3860.1413, 587.375) -> (-3720.8617, 598.0823) centre (-3860.1413, 1498.6) ccw
  line L7 (-3860.1413, 606.425) -> (-4241.8, 606.425)
  arc A2 (-3860.1413, 606.425) -> (-3723.7735, 616.9084) centre (-3860.1413, 1498.6) ccw
  dimension "d110" = -250.825
  dimension "d111" = -231.775
  dimension "d112" = 250.825
  dimension "d113" = 231.775
extrude "Extrude15" add sketch "Sketch13" along normal blind 0.0279 contours L0 L2 L4 L5
extrude "Extrude16" add sketch "Sketch13" along normal blind 0.0279 contours L0 L2 L6 A1 L7 A2
